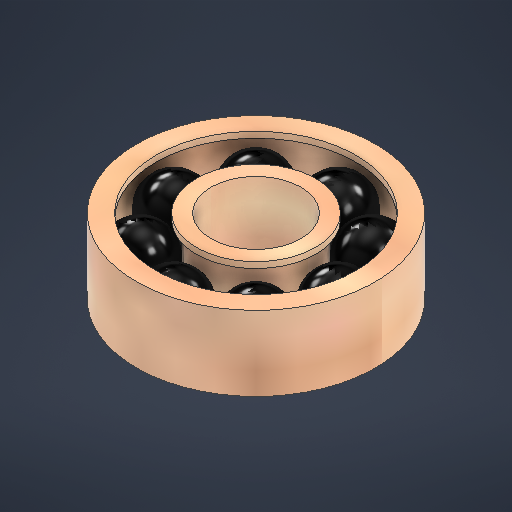
# Autodesk Inventor part: Bearing
Saved by Autodesk Inventor 2026.1 (Build 301233000, 233)
## iProperties
Created: 2026-07-13
Part Number: Bearing
Material: Generic
Document SubType Name: Modeling
Designer: ankit
Density: 1 g/cm^3
Appearance: Default
Author: ankit
Autodesk Inventor part; units mm, degrees
ref_plane "YZ Plane" through (0, 0, 0) normal (1, 0, 0) x (0, 1, 0)
ref_plane "XZ Plane" through (0, 0, 0) normal (0, 1, 0) x (-1, 0, 0)
ref_plane "XY Plane" through (0, 0, 0) normal (0, 0, 1) x (1, 0, 0)
sketch "Sketch1" plane through (0, 0, 0) normal (0, 1, 0) x (-1, 0, 0)
  circle A0 centre (0, 0) radius 4
  circle A1 centre (0, 0) radius 1.5
  line L0 (1.5, 0) -> (4, 0)
  circle A2 centre (0, 0) radius 1.75
  circle A3 centre (0, 0) radius 3.75
  arc A4 (3.75, 0) -> (1.75, 0) centre (2.75, 0) ccw
  point P0 (1.75, 0)
  dimension "d0" = 8
  dimension "d1" = 3
  dimension "d2" = 3.5
  dimension "d3" = 7.5
  constraints: 4 coincident, 4 horizontal alignment, 2 end point, 2 point on circle, 1 centre point, 1 horizontal, 1 midpoint, 8 other
revolve "Revolution1" add sketch "Sketch1" angle 360 about axis through (-1.5, 0, 0) along (-1, 0, 0) contours L0 A4
extrude "Extrusion1" add sketch "Sketch1" along normal mid plane 2.5 contours A0 | A2
pattern_circular "Circular Pattern1" count 8 over 360 about axis through (0, -10, 0) along (0, 1, 0) of "Revolution1"
sketch "Sketch2" plane through (0, -1.25, 0) normal (0, -1, 0) x (1, 0, 0)
  circle A0 centre (0, 0) radius 3.35
  circle A1 centre (0, 0) radius 3.75
  circle A2 centre (0, 0) radius 1.75
  circle A3 centre (0, 0) radius 2
  dimension "d10" = 6.7
  dimension "d13" = 4
  constraints: 6 coincident, 4 centre point
  measures "d10" diameter of A0
  measures "d13" diameter of A3
extrude "Extrusion2" add sketch "Sketch2" against normal blind 0.2
mirror "Mirror1" about plane through (0, 0, 0) normal (0, 1, 0) of "Extrusion2"
body "Solid1"
